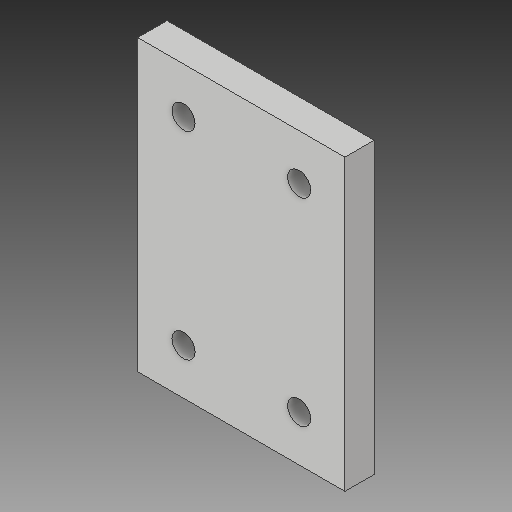
# Autodesk Inventor part: Part3
Saved by Autodesk Inventor 2019 (Build 230136000, 136)
## iProperties
Created: 2019-05-13
Part Number: Part3
Material: Generic
Document SubType Name: Modeling
Designer: Alex Jones
Density: 1 g/cm^3
Appearance: Default
Mass: 17.3097 g
Surface Area: 72.1484 cm^2
Volume: 17.3097 cm^3
Author: Alex Jones
Autodesk Inventor part; units mm, degrees
ref_plane "YZ Plane" through (0, 0, 0) normal (1, 0, 0) x (0, 1, 0)
ref_plane "XZ Plane" through (0, 0, 0) normal (0, 1, 0) x (-1, 0, 0)
ref_plane "XY Plane" through (0, 0, 0) normal (0, 0, 1) x (1, 0, 0)
sketch "Sketch1" plane through (0, 0, 0) normal (0, 0, 1) x (1, 0, 0)
  circle A0 centre (-144.8611, 31.4) radius 2.5 projected
  circle A1 centre (-144.8611, 31.4) radius 9.9 construction
  circle A2 centre (-169.8611, 31.4) radius 2.5 projected
  circle A3 centre (-169.8611, 31.4) radius 9.9 construction
  circle A4 centre (-169.8611, -11.4) radius 2.5 projected
  circle A5 centre (-169.8611, -11.4) radius 9.9 construction
  circle A6 centre (-144.8611, -11.4) radius 2.5 projected
  circle A7 centre (-144.8611, -11.4) radius 9.9 construction
  line L0 (-144.8611, 31.4) -> (-169.8611, 31.4) construction
  line L1 (-169.8611, 31.4) -> (-169.8611, -11.4) construction
  line L2 (-169.8611, -11.4) -> (-144.8611, -11.4) construction
  line L3 (-144.8611, -11.4) -> (-144.8611, 31.4) construction
  line L4 (-134.9611, 41.3) -> (-179.7611, 41.3)
  line L5 (-179.7611, 41.3) -> (-179.7611, -21.3)
  line L6 (-179.7611, -21.3) -> (-134.9611, -21.3)
  line L7 (-134.9611, -21.3) -> (-134.9611, 41.3)
  point P0 (0, 0)
  constraints: 16 end point, 4 parallel, 2 perpendicular, 1 horizontal, 1 tangent, 3 other
extrude "Extrusion1" add sketch "Sketch1" along normal blind 6.35
body "Solid1"
